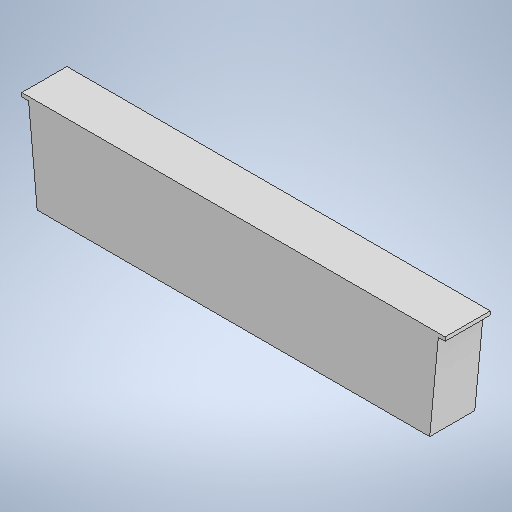
# Autodesk Inventor part: Lid_Divider
Saved by Autodesk Inventor 2025 (Build 290162010, 162A)
## iProperties
Created: 2024-10-17
Part Number: Lid_Divider
Material: Generic
Document SubType Name: Modeling
Designer: vncnt
Density: 1 g/cm^3
Appearance: Default
Author: vncnt
Autodesk Inventor part; units mm, degrees
ref_plane "YZ Plane" through (0, 0, 0) normal (1, 0, 0) x (0, 1, 0)
ref_plane "XZ Plane" through (0, 0, 0) normal (0, 1, 0) x (-1, 0, 0)
ref_plane "XY Plane" through (0, 0, 0) normal (0, 0, 1) x (1, 0, 0)
sketch "Sketch1" plane through (0, 0, 0) normal (0, 0, 1) x (1, 0, 0)
  line L0 (-110.49, 25.4) -> (110.49, 25.4)
  line L1 (110.49, 25.4) -> (110.49, -25.4)
  line L2 (110.49, -25.4) -> (-110.49, -25.4)
  line L3 (-110.49, -25.4) -> (-110.49, 25.4)
  line L4 (-110.49, 25.4) -> (110.49, -25.4) construction
  line L5 (110.49, 25.4) -> (-110.49, -25.4) construction
  line L6 (0, 25.4) -> (115.316, 25.4)
  line L7 (115.316, 25.4) -> (110.49, -25.4)
  line L8 (0, 25.4) -> (-115.316, 25.4)
  line L9 (-115.316, 25.4) -> (-110.49, -25.4)
  line L10 (119.1514, 25.4) -> (-119.1514, 25.4)
  line L11 (-119.1514, 25.4) -> (-119.1514, 27.5463)
  line L12 (-119.1514, 27.5463) -> (119.1514, 27.5463)
  line L13 (119.1514, 27.5463) -> (119.1514, 25.4)
  point P0 (0, 0)
  point P1 (0, 27.5463)
  point P2 (110.49, 25.4)
  point P3 (110.49, 25.4)
  dimension "d0" = 220.98
  dimension "d1" = 50.8
  dimension "d2" = 115.316
  dimension "d3" = 115.316
  dimension "d10" = 2.1463
  dimension "d11" = 238.3028
  constraints: 28 end point, 4 midpoint, 3 horizontal, 3 parallel, 2 perpendicular, 2 point on line
  measures "d0" distance of L1.end L2.end
  measures "d1" distance of L0.end L1.end
  measures "d2" distance of L6.start L6.end
  measures "d3" distance of L6.start L8.end
  measures "d10" distance of L12.end L10.start
  measures "d11" distance of L11.end L12.end
extrude "Extrusion1" add sketch "Sketch1" along normal blind 25.4
sketch "Sketch2" plane through (0, 0, 25.4) normal (0, 0, 1) x (1, 0, 0)
  line L0 (-120.0424, 48.8596) -> (122.5706, 48.8596)
  line L1 (122.5706, 48.8596) -> (122.5706, -0.3726)
  line L2 (122.5706, -0.3726) -> (-120.0424, -0.3726)
  line L3 (-120.0424, -0.3726) -> (-120.0424, 48.8596)
  point P0 (0, 0)
  constraints: 8 end point, 2 parallel, 1 horizontal, 1 perpendicular
extrude "Extrusion2" [suppressed]
body "Solid1"
